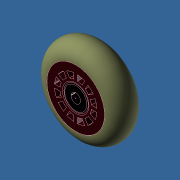
# Autodesk Inventor part: Wheel
Saved by Autodesk Inventor 2018 (Build 220112000, 112)
## iProperties
Created: 2018-02-14
Part Number: Wheel
Material: Rubber
Document SubType Name: Modeling
Designer: Cole
Density: 0.93 g/cm^3
Appearance: Smooth - Medium Gray
Author: Cole
Autodesk Inventor part; units mm, degrees
ref_plane "YZ Plane" through (0, 0, 0) normal (1, 0, 0) x (0, 1, 0)
ref_plane "XZ Plane" through (0, 0, 0) normal (0, 1, 0) x (-1, 0, 0)
ref_plane "XY Plane" through (0, 0, 0) normal (0, 0, 1) x (1, 0, 0)
sketch "Sketch1" plane through (0, 0, 0) normal (0, 0, 1) x (1, 0, 0)
  circle A0 centre (0, 0) radius 36.83
  dimension "d0" = 73.66
  constraints: 1 centre point, 1 coincident
  measures "d0" diameter of A0
extrude "Extrusion1" add sketch "Sketch1" along normal blind 24.384
full round fillet "Fillet1" first side at (7.2727, -4.1989, 24.384) centre faces at (36.7193, -2.854, 16.256) second side at (7.2727, -4.1989, 0)
sketch "Sketch3" plane through (0, 0, 24.384) normal (0, 0, 1) x (1, 0, 0)
  circle A0 centre (0, 0) radius 4.064
  dimension "d6" = 8.128
  constraints: 1 centre point, 1 coincident
  measures "d6" diameter of A0
extrude "Extrusion3" cut sketch "Sketch3" against normal blind 25.4
sketch "Sketch4" plane through (0, 0, 24.384) normal (0, 0, 1) x (1, 0, 0)
  circle A0 centre (0, 0) radius 36.83 projected
  line L0 (0, 0) -> (31.595, 0) construction
  line L1 (18.1479, 1.524) -> (13.3755, 1.524)
  line L2 (18.1479, -1.524) -> (13.3755, -1.524)
  line L3 (14.9546, 10.3938) -> (10.8215, 8.0076)
  line L4 (16.4786, 7.7541) -> (12.3455, 5.3679)
  line L5 (7.7541, 16.4786) -> (5.3679, 12.3455)
  line L6 (10.3938, 14.9546) -> (8.0076, 10.8215)
  line L7 (-1.524, 18.1479) -> (-1.524, 13.3755)
  line L8 (1.524, 18.1479) -> (1.524, 13.3755)
  line L9 (-10.3938, 14.9546) -> (-8.0076, 10.8215)
  line L10 (-7.7541, 16.4786) -> (-5.3679, 12.3455)
  line L11 (-16.4786, 7.7541) -> (-12.3455, 5.3679)
  line L12 (-14.9546, 10.3938) -> (-10.8215, 8.0076)
  line L13 (-18.1479, -1.524) -> (-13.3755, -1.524)
  line L14 (-18.1479, 1.524) -> (-13.3755, 1.524)
  line L15 (-14.9546, -10.3938) -> (-10.8215, -8.0076)
  line L16 (-16.4786, -7.7541) -> (-12.3455, -5.3679)
  line L17 (-7.7541, -16.4786) -> (-5.3679, -12.3455)
  line L18 (-10.3938, -14.9546) -> (-8.0076, -10.8215)
  line L19 (1.524, -18.1479) -> (1.524, -13.3755)
  line L20 (-1.524, -18.1479) -> (-1.524, -13.3755)
  line L21 (10.3938, -14.9546) -> (8.0076, -10.8215)
  line L22 (7.7541, -16.4786) -> (5.3679, -12.3455)
  line L23 (16.4786, -7.7541) -> (12.3455, -5.3679)
  line L24 (14.9546, -10.3938) -> (10.8215, -8.0076)
  arc A1 (14.9546, 10.3938) -> (10.3938, 14.9546) centre (0, 0) ccw
  arc A2 (10.8215, 8.0076) -> (8.0076, 10.8215) centre (0, 0) ccw
  arc A3 (13.3755, 1.524) -> (12.3455, 5.3679) centre (0, 0) ccw
  arc A4 (18.1479, 1.524) -> (16.4786, 7.7541) centre (0, 0) ccw
  arc A5 (16.4786, -7.7541) -> (18.1479, -1.524) centre (0, 0) ccw
  arc A6 (12.3455, -5.3679) -> (13.3755, -1.524) centre (0, 0) ccw
  arc A7 (8.0076, -10.8215) -> (10.8215, -8.0076) centre (0, 0) ccw
  arc A8 (10.3938, -14.9546) -> (14.9546, -10.3938) centre (0, 0) ccw
  arc A9 (1.524, -18.1479) -> (7.7541, -16.4786) centre (0, 0) ccw
  arc A10 (1.524, -13.3755) -> (5.3679, -12.3455) centre (0, 0) ccw
  arc A11 (-7.7541, -16.4786) -> (-1.524, -18.1479) centre (0, 0) ccw
  arc A12 (-5.3679, -12.3455) -> (-1.524, -13.3755) centre (0, 0) ccw
  arc A13 (-14.9546, -10.3938) -> (-10.3938, -14.9546) centre (0, 0) ccw
  arc A14 (-10.8215, -8.0076) -> (-8.0076, -10.8215) centre (0, 0) ccw
  arc A15 (-18.1479, -1.524) -> (-16.4786, -7.7541) centre (0, 0) ccw
  arc A16 (-13.3755, -1.524) -> (-12.3455, -5.3679) centre (0, 0) ccw
  arc A17 (-16.4786, 7.7541) -> (-18.1479, 1.524) centre (0, 0) ccw
  arc A18 (-12.3455, 5.3679) -> (-13.3755, 1.524) centre (0, 0) ccw
  arc A19 (-10.3938, 14.9546) -> (-14.9546, 10.3938) centre (0, 0) ccw
  arc A20 (-8.0076, 10.8215) -> (-10.8215, 8.0076) centre (0, 0) ccw
  arc A21 (7.7541, 16.4786) -> (1.524, 18.1479) centre (0, 0) ccw
  arc A22 (-1.524, 18.1479) -> (-7.7541, 16.4786) centre (0, 0) ccw
  arc A23 (5.3679, 12.3455) -> (1.524, 13.3755) centre (0, 0) ccw
  arc A24 (-1.524, 13.3755) -> (-5.3679, 12.3455) centre (0, 0) ccw
  dimension "d11" = 1.524
  dimension "d12" = 1.524
  dimension "d15" = 360
  constraints: 50 end point, 48 point on circle, 24 centre point, 2 coincident, 2 horizontal, 1 parallel, 73 other
  measures "d11" distance between parallel lines of L0 L1
  measures "d12" distance between parallel lines of L0 L2
extrude "Extrusion4" cut sketch "Sketch4" against normal blind 25.4 contours L1 A3 L4 A4 | A5 L23 A6 L2 | L3 A2 L6 A1 | L5 A23 L8 A21 | L7 A24 L10 A22 | L9 A20 L12 A19 | L11 A18 L14 A17 | L13 A16 L16 A15 | L15 A14 L18 A13 | L17 A12 L20 A11 | L19 A10 L22 A9 | L21 A7 L24 A8
sketch "Sketch5" plane through (0, 0, 24.384) normal (0, 0, 1) x (1, 0, 0)
  circle A0 centre (0, 0) radius 10.414
  circle A1 centre (0, 0) radius 4.064 projected
  dimension "d19" = 6.35
  constraints: 1 centre point, 1 coincident
  measures "d19" radial gap between concentric circles of A1 A0
sketch "Sketch6" plane through (0, 0, 0) normal (0, 0, -1) x (-1, 0, 0)
  circle A0 centre (0, 0) radius 10.414
  circle A1 centre (0, 0) radius 4.064 projected
  dimension "d20" = 6.35
  constraints: 1 centre point, 1 coincident
  measures "d20" radial gap between concentric circles of A1 A0
ref_plane "Work Plane1" through (0, 0, 0) normal (-0.5, -0.8660254, 0) x (0.8660254, -0.5, 0)
sketch "Sketch7" plane through (0, 0, 0) normal (-0.5, -0.8660254, 0) x (0.8660254, -0.5, 0)
  line L0 (-10.414, 0) -> (10.414, 0) projected
  line L1 (0, 24.0485) -> (0, 17.0458)
  line L2 (10.1174, 24.4001) -> (10.414, 24.0485)
  line L3 (10.414, 24.0485) -> (10.8307, 24.4001)
  line L4 (10.8307, 24.4001) -> (10.1174, 24.4001)
  line L5 (-10.414, 0) -> (10.414, 0)
  line L6 (0, 24.0485) -> (0, 17.0458)
  line L7 (10.1174, 24.4001) -> (10.414, 24.0485)
  line L8 (10.414, 24.0485) -> (10.8307, 24.4001)
  line L9 (10.8307, 24.4001) -> (10.1174, 24.4001)
  point P0 (0, 0)
  point P1 (0, 0)
  constraints: 18 end point, 2 horizontal, 2 perpendicular, 2 vertical
revolve "Revolution1" cut sketch "Sketch7" angle 360 about axis through (0, 0, 24.0485) along (0, 0, -1)
fillet "Fillet2" radius 1.524 2 edges at (-8.7737, 5.0655, 24.384) (-9.3631, 5.4058, 24.384)
ref_plane "Work Plane2" through (0, 0, 12.192) normal (0, 0, -1) x (-1, 0, 0)
sketch "Sketch8" plane through (0, 0, 12.192) normal (0, 0, -1) x (-1, 0, 0)
  line L0 (-39.5252, -39.6083) -> (38.5017, -39.6083)
  line L1 (38.5017, -39.6083) -> (38.5017, 38.9039)
  line L2 (38.5017, 38.9039) -> (-39.5252, 38.9039)
  line L3 (-39.5252, 38.9039) -> (-39.5252, -39.6083)
  point P0 (0, 0)
  constraints: 8 end point, 2 parallel, 1 horizontal, 1 perpendicular
extrude "Extrusion5" cut sketch "Sketch8" along normal blind 31.75
mirror "Mirror1" about plane through (0, 0, 12.192) normal (0, 0, -1)
sketch "Sketch9" plane through (0, 0, 24.384) normal (0, 0, 1) x (1, 0, 0)
  point P0 (0, 0)
  point P1 (0, 0)
  constraints: 1 coincident
ref_plane "Work Plane3" through (0, 0, 24.384) normal (1, 0, 0) x (0, 0, -1)
sketch "Sketch10" plane through (0, 0, 24.384) normal (1, 0, 0) x (0, 0, -1)
  line L0 (-0.0067, 24.6498) -> (-0.0067, 24.6234)
  line L1 (-0.0067, 24.6234) -> (0.0112, 24.6332)
  line L2 (0.0112, 24.6332) -> (-0.0067, 24.6498)
  line L3 (-1.2724, 0) -> (3.1027, 0)
  line L4 (24.384, -24.638) -> (24.384, 24.638) projected
  line L5 (0, -24.638) -> (0, 24.638) projected
  arc A0 (24.384, 24.638) -> (0, 24.638) centre (12.192, 24.638) ccw projected
  line L6 (12.192, 36.83) -> (12.192, -36.83)
  arc A1 (0, -24.638) -> (24.384, -24.638) centre (12.192, -24.638) ccw projected
  line L7 (24.3907, 24.6498) -> (24.3907, 24.6234)
  line L8 (24.3907, 24.6234) -> (24.3728, 24.6332)
  line L9 (24.3728, 24.6332) -> (24.3907, 24.6498)
  line L10 (25.6564, 0) -> (21.2813, 0)
  line L11 (24.384, -24.638) -> (24.384, 24.638)
  point P0 (24.384, 0)
  constraints: 20 end point, 9 symmetric about line, 2 point on circle, 2 vertical, 1 horizontal
revolve "Revolution2" cut sketch "Sketch10" angle 360 about axis through (0, 0, 25.6564) along (0, 0, -1) contours L2 A0 L5 L1 L0 | L2 L1 L5 A0
body "Solid1"
